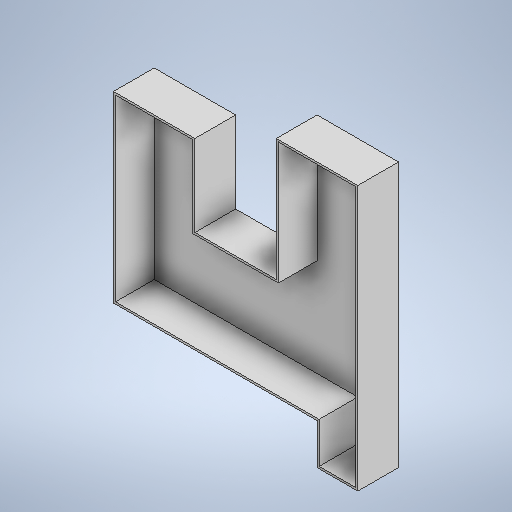
# Autodesk Inventor part: Spacer
Saved by Autodesk Inventor 2025.2 (Build 292293000, 293)
## iProperties
Created: 2025-02-09
Part Number: Spacer
Material: Generic
Document SubType Name: Modeling
Designer: kenne
Density: 1 g/cm^3
Appearance: Default
Author: kenne
## iProperties of the stored document Spacer_3DPrint.ipt
Created: 2025-02-09
Part Number: Spacer_3DPrint
Material: Generic
Document SubType Name: Modeling
Designer: kenne
Density: 1 g/cm^3
Appearance: Default
Author: kenne
Autodesk Inventor part; units mm, degrees
ref_plane "YZ Plane" through (0, 0, 0) normal (1, 0, 0) x (0, 1, 0)
ref_plane "XZ Plane" through (0, 0, 0) normal (0, 1, 0) x (-1, 0, 0)
ref_plane "XY Plane" through (0, 0, 0) normal (0, 0, 1) x (1, 0, 0)
sketch "Sketch1" plane through (0, 0, 0) normal (0, 0, 1) x (1, 0, 0)
  line L0 (0, 2.4004) -> (60, 2.4004) construction
  line L1 (-60, 0) -> (60, 0) construction
  line L2 (-60, 0) -> (-60, 20) construction
  line L3 (-60, 20) -> (40, 20)
  line L4 (40, 20) -> (40, 0)
  line L5 (40, 0) -> (60, 0)
  line L6 (60, 0) -> (60, 130)
  line L7 (75, 0) -> (75, 70) construction
  line L8 (-60, 20) -> (-60, 110)
  line L9 (-60, 110) -> (-20, 110)
  line L10 (-20, 110) -> (-20, 70)
  line L11 (-20, 70) -> (20, 70)
  line L12 (20, 70) -> (20, 130)
  line L13 (20, 130) -> (60, 130)
  point P0 (0, 0)
  dimension "d2" = 120
  dimension "d3" = 20
  dimension "d4" = 100
  dimension "d5" = 20
  dimension "d6" = 20
  dimension "d7" = 130
  dimension "d8" = 70
  dimension "d9" = 90
  dimension "d10" = 40
  dimension "d11" = 40
  constraints: 28 end point, 4 horizontal, 4 vertical, 3 perpendicular, 1 collinear, 1 point on line
  measures "d2" distance of L1.start L1.end
  measures "d3" distance of L1.start L2.end
  measures "d4" distance of L2.end L3.end
  measures "d5" distance of L3.end L4.end
  measures "d6" distance of L4.end L1.end
  measures "d7" distance of L1.end L6.end
  measures "d8" distance of L7.start L7.end
  measures "d9" distance of L2.end L8.end
  measures "d10" distance of L8.end L9.end
  measures "d11" distance of L10.end L11.end
extrude "Extrusion1" add sketch "Sketch1" along normal blind 20
shell "Shell1" thickness 1 removed faces 1 at (-13.3333, 36.6667, 20)
body "Solid1"
